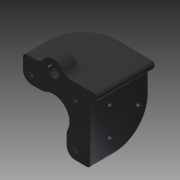
# Autodesk Inventor part: Z_bottom
Saved by Autodesk Inventor 2013 (Build 170138000, 138)
## iProperties
Created: 2014-01-18
Part Number: Z_bottom
Material: Generic
Document SubType Name: Modeling
Designer: Masta
Density: 1 g/cm^3
Author: Masta
Autodesk Inventor part; units mm, degrees
note: some values were not read from the file. Chosen so that the rebuilt part matches the saved one: sketch regions of "Extrusion1".
ref_plane "YZ Plane" through (0, 0, 0) normal (1, 0, 0) x (0, 1, 0)
ref_plane "XZ Plane" through (0, 0, 0) normal (0, 1, 0) x (-1, 0, 0)
ref_plane "XY Plane" through (0, 0, 0) normal (0, 0, 1) x (1, 0, 0)
sketch "Sketch1" plane through (0, 0, 0) normal (0, 1, 0) x (-1, 0, 0)
  circle A0 centre (0, 0) radius 11.5
  line L0 (21.25, 21.25) -> (-21.25, 21.25)
  line L1 (-21.25, 21.25) -> (-21.25, -21.25)
  line L2 (-21.25, -21.25) -> (-9.5, -21.25)
  line L3 (21.25, -21.25) -> (21.25, 9.5) construction
  line L4 (21.25, 21.25) -> (-21.25, -21.25) construction
  line L5 (-21.25, 21.25) -> (21.25, -21.25) construction
  line L6 (15.5, 15.5) -> (-15.5, 15.5) construction
  line L7 (-15.5, 15.5) -> (-15.5, -15.5) construction
  line L8 (-15.5, -15.5) -> (15.5, -15.5) construction
  line L9 (15.5, -15.5) -> (15.5, 15.5) construction
  line L10 (15.5, 15.5) -> (-15.5, -15.5) construction
  line L11 (-15.5, 15.5) -> (15.5, -15.5) construction
  line L12 (-21.25, -21.25) -> (-26.25, -21.25)
  line L13 (-26.25, -21.25) -> (-26.25, 21.25)
  line L14 (21.25, 26.25) -> (21.25, 21.25)
  line L15 (-9.5, -21.25) -> (-9.5, -6.4807)
  line L16 (6.4807, 9.5) -> (21.25, 9.5)
  line L17 (-9.5, -21.25) -> (21.25, -21.25) construction
  line L18 (21.25, 9.5) -> (21.25, 21.25)
  line L19 (-31.25, 26.25) -> (-31.25, 21.25)
  line L20 (-31.25, 21.25) -> (-26.25, 21.25)
  line L21 (21.25, 26.25) -> (-31.25, 26.25)
  circle A1 centre (0, 25) radius 4
  line L22 (0, 0) -> (0, 25) construction
  circle A2 centre (0, 25) radius 8
  arc A3 (7.9017, 26.25) -> (-7.9017, 26.25) centre (0, 25) ccw
  line L23 (-7.9017, 26.25) -> (7.9017, 26.25)
  dimension "d0" = 23
  dimension "d1" = 42.5
  dimension "d2" = 42.5
  dimension "d3" = 31
  dimension "d4" = 31
  dimension "d5" = 5
  dimension "d6" = 5
  dimension "d7" = 6
  dimension "d8" = 6
  dimension "d10" = 5
  dimension "d11" = 25
  dimension "d12" = 8
  dimension "d13" = 4
  constraints: 48 end point, 10 perpendicular, 8 parallel, 6 coincident, 4 midpoint, 4 point on circle, 3 centre point, 2 collinear, 2 horizontal, 2 point on line, 3 other
  measures "d0" diameter of A0
  measures "d1" distance of L3.start L1.end
  measures "d2" distance of L1.end L0.end
  measures "d3" distance of L8.end L7.end
  measures "d4" distance of L7.end L6.end
  measures "d5" distance of L1.end L12.end
  measures "d6" distance of L14.start L0.start
  measures "d7" distance between parallel lines of L16 L6
  measures "d8" distance between parallel lines of L7 L15
  measures "d10" distance of L19.end L13.end
  measures "d11" distance of L22.start L22.end
  measures "d12" diameter of A1
  measures "d13" radius of A1
extrude "Extrusion1" add sketch "Sketch1" against normal blind 5 contours A0 L15 L2 L1 L0 A2 L18 L16 | L0 A2 L21 L14 | L12 L13 L20 L19 L21 A2 L0 L1 | A2 L0 A1 | L0 A1 L21 A2 | A1 L0 | L0 A1 L21 | A2 L21 A1 L0 | L21 A1 A2
extrude "Extrusion2" cut sketch "Sketch1" against normal up to next contours A1 L0 | L0 A1 L21 | L21 A1
extrude "Extrusion3" add sketch "Sketch1" along normal blind 37 contours L0 A2 L21 L14 | L12 L13 L20 L19 L21 A2 L0 L1 | L0 A1 L21 A2 | L0 A1 L21 | A2 L21 A1 L0
hole "Hole1" at (15.5, 0, 15.5) at (15.5, 0, -15.5) at (-15.5, 0, 15.5) direction (0, -1, 0) diameter 3.2 end through all
extrude "Extrusion4" add sketch "Sketch1" along normal blind 5 contours L21 A1 A2 | L21 A1
extrude "Extrusion5" add sketch "Sketch1" along normal blind 0.3 contours A1 L0 | L0 A1 L21 | L21 A1
fillet "Fillet2" radius 6 6 edges at (9.5, -2.5, -21.25) (-21.25, -2.5, 9.5) (-6.4807, -2.5, 9.5) (9.5, -2.5, -6.4807) (7.9017, 0, 26.25) (-7.9017, 0, 26.25)
sketch "Sketch2" plane through (21.25, 0, 21.25) normal (-1, 0, 0) x (0, 0, 1)
  line L0 (0, 0) -> (-42.5, 0) projected
  line L1 (0, 0) -> (0, 37) projected
  line L2 (-42.5, 0) -> (-42.5, 37) projected
  line L3 (-30, 9) -> (-10, 9) construction
  line L4 (-20, 9) -> (-20, 29) construction
  circle A0 centre (-20, 29) radius 4
  circle A1 centre (-30, 9) radius 4
  circle A2 centre (-10, 9) radius 4
  point P0 (-21.25, 0)
  dimension "d34" = 20
  dimension "d36" = 20
  dimension "d37" = 10
  dimension "d38" = 9
  dimension "d46" = 8
  constraints: 6 coincident, 4 end point, 3 centre point, 2 equal radius, 2 perpendicular, 1 midpoint
  measures "d34" distance of L3.start L3.end
  measures "d36" distance of L4.start L4.end
  measures "d37" distance from line of L1 L3.end
  measures "d38" distance between parallel lines of L0 L3
  measures "d46" diameter of A0
hole "Hole2" at (21.25, 9, -8.75) at (21.25, 29, 1.25) at (21.25, 9, 11.25) direction (1, 0, 0) diameter 3.2 end through all
extrude "Extrusion6" cut sketch "Sketch2" against normal blind 2.7
fillet "Fillet4" radius 25 2 edges at (23.75, 37, -21.25) (-21.25, 37, 23.75)
fillet "Fillet3" radius 2.5 9 edges at (-21.25, 3.5, 26.25) (31.25, 16, 26.25) (31.25, 16, 21.25) (26.25, 3.5, -21.25) (21.25, 6, -21.25) (-21.25, 6, 21.25) (21.25, 18.5, 21.25) (28.75, 37, 21.25) (31.25, 37, 23.75)
fillet "Fillet5" radius 1 3 edges at (21.25, 9, 7.25) (21.25, 9, -12.75) (21.25, 29, -2.75)
body "Solid1"
